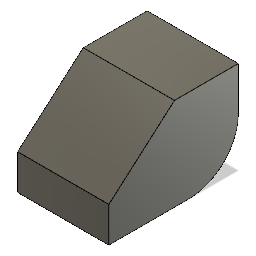
5.1 planes (Autodesk Fusion 360 design; units mm, degrees)
Autodesk Fusion 360 part; units mm, degrees
sketch "Sketch1" plane through (0, 0, 0) normal (1, 0, 0) x (0, 0, -1)
  line L0 (0, 0) -> (0, 45.7222)
  line L1 (0, 45.7222) -> (-31.5831, 45.7222)
  line L2 (-31.5831, 45.7222) -> (-63.9629, 17.487)
  line L3 (-63.9629, 17.487) -> (-63.9629, 0)
  line L4 (-63.9629, 0) -> (0, 0)
extrude "Extrude1" add sketch "Sketch1" along normal blind 45.086
fillet "Fillet1" radius 24.459 1 edges at (22.543, 0, 0)
